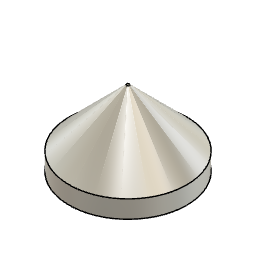
electrode coating tool v7 (Autodesk Fusion 360 design; units mm, degrees)
Autodesk Fusion 360 part; units mm, degrees
sketch "Sketch1" plane through (0, 0, 0) normal (0, 0, 1) x (1, 0, 0)
  line L0 (0, 0) -> (0, 9.5)
  line L1 (0, 9.5) -> (3.5, 6)
  line L2 (3.5, 6) -> (3.5, 5)
  line L3 (3.5, 5) -> (12.5, 5)
  line L4 (12.5, 5) -> (12.5, 0)
  line L5 (12.5, 0) -> (0, 0)
  line L6 (0, 9.475) -> (0.025, 9.475)
  line L7 (12.5, 8) -> (12.5, 6)
  line L8 (12.5, 6) -> (4, 6)
  line L9 (4, 6) -> (4, 8)
  line L10 (4, 8) -> (12.5, 8)
  line L11 (1, 8.5) -> (1, 8.2)
  line L12 (1, 8.2) -> (0, 8.2)
  line L13 (1, 8.3) -> (1.2, 8.3)
  dimension "d1" = 12.5
  dimension "d2" = 3.5
  dimension "d3" = 45
  dimension "d4" = 1
  dimension "d5" = 5
  dimension "d7" = 0.025
  dimension "d8" = 8.5
  dimension "d10" = 2
  dimension "d20" = 1
  dimension "d21" = 1.3
  dimension "d22" = 0.1
  constraint coincident L0.start L5.end
  constraint vertical L0
  constraint parallel L0 L2
  constraint perpendicular L2 L3
  constraint perpendicular L3 L4
  constraint perpendicular L0 L5
  constraint coincident L0 L6.start
  constraint coincident L1 L6.end
  constraint perpendicular L0 L6
  constraint vertical L7
  constraint perpendicular L7 L8
  constraint perpendicular L8 L9
  constraint horizontal L10
  constraint coincident L1.end L8
  constraint collinear L4 L7
  constraint coincident L1 L11.start
  constraint vertical L11
  constraint coincident L0 L12.end
  constraint perpendicular L0 L12
  constraint coincident L11 L13.start
  constraint coincident L1 L13.end
  constraint perpendicular L11 L13
  measures "d1" distance of L4.end L0.start
  measures "d2" distance of L0 L2
  measures "d3" angle of L0 L1
  measures "d4" distance of L1.end L2.end
  measures "d5" distance of L3.end L4.end
  measures "d7" distance of L6.start L6.end
  measures "d8" distance of L7.start L9.end
  measures "d10" distance of L7.start L7.end
  measures "d20" distance of L0 L11
  measures "d21" distance of L0.end L12
  measures "d22" distance of L12 L13
revolve "Revolve1" add sketch "Sketch1" angle 360 about axis through (0, 0, 0) along (0, 1, 0) contours L0 L1 L2 L3 L4 L5 L11 L12 L13 | L7 L8 L9 L10 makes body 1 at (-3.3879, 0, 0.621) makes body 2 at (9.6201, 8, 0.621)
sketch "Sketch3" plane through (0, 8, 0) normal (0, 1, 0) x (-1, 0, 0)
  circle A0 centre (0, 0) radius 4
  circle A1 centre (0, 0) radius 12.5
  circle A2 centre (0, 0) radius 12.5
  line L0 (1.6, -12.3972) -> (1.6, -10.8972)
  arc A3 (1.6, -10.8972) -> (-1.6, -10.8972) centre (0, -10.8972) ccw
  line L1 (-1.6, -10.8972) -> (-1.6, -12.3972)
  dimension "d11" = 1.6
  dimension "d12" = 1.5
  constraint coincident A2 L0.start
  constraint vertical L0
  constraint tangent L0 A3
  constraint coincident A2 L1.end
  constraint tangent A3 L1
  constraint parallel L0 L1
  constraint vertical A0.centre A3.centre
  measures "d11" radius of A3
  measures "d12" vertical distance of A3.centre L1.end
extrude "Extrude1" cut sketch "Sketch3" against normal blind 2 contours A1 A2 L0 A3 L1 picked at (-0.1782, -11.4276) bodies 2
hole "Hole1" at (0, 8, -10.8972) direction (0, -1, 0) diameter 1.623 depth 10 tip angle 118 bodies 1
thread "Thread1" "ISO Metric profile 2.0 M2x0.4 6H" thread offset 0 thread depth 10
pattern_circular "C-Pattern1" count 3 over 360 about axis through (0, 1.75, 0) along (0, 1, 0) of "Extrude1", "Hole1"
revolve "Revolve2" add sketch "Sketch1" angle 360 about axis through (0, 0, 0) along (0, 1, 0) separate body contours L0 L1 L6 L11 L12 makes body 3
move_face "OffsetFaces1" offset -0.05 1 faces at (0.9988, 8.2667, 0.0498) on bodies 1
copy_body "Body->Comp1" bodies 1 removing the originals makes body 4 in component "form"
copy_body "Body->Comp2" bodies 2 removing the originals makes body 5 in component "clamp"
copy_body "Body->Comp3" bodies 3 removing the originals makes body 6 in component "thorn"
component "form" placed x (1, 0, 0) y (0, 1, 0) z (0, 0, 1) at (0, 0, 0)
component "clamp" placed x (1, 0, 0) y (0, 1, 0) z (0, 0, 1) at (0, 0, 0)
component "thorn" placed x (1, 0, 0) y (0, 1, 0) z (0, 0, 1) at (0, 0, 0)
named bodies: "form", "clamp", "thorn"
